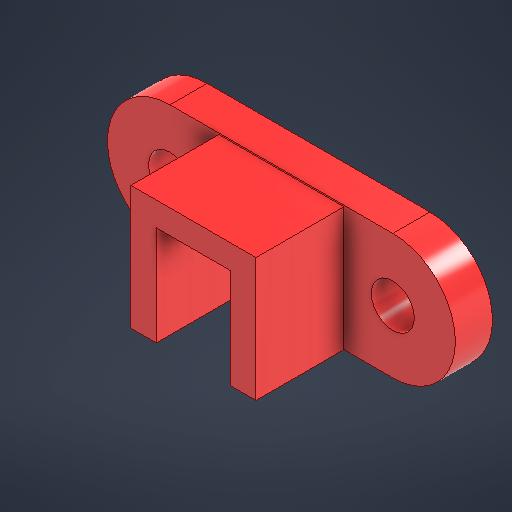
# Autodesk Inventor part: PART 7
Saved by Autodesk Inventor 2026.2 (Build 302298000, 298)
## iProperties
Created: 2026-03-26
Part Number: PART 7
Material: Nylon 6/6
Document SubType Name: Modeling
Designer: LENOVO
Density: 1.13 g/cm^3
Appearance: Light Red
Author: LENOVO
Autodesk Inventor part; units mm, degrees
ref_plane "YZ Plane" through (0, 0, 0) normal (1, 0, 0) x (0, 1, 0)
sketch "Sketch1" plane through (0, 0, 0) normal (0, 0, 1) x (1, 0, 0)
  point P0 (0, 0)
sketch "Sketch2" plane through (0, 0, 0) normal (0, 0, 1) x (1, 0, 0)
  line L0 (-53.7332, 0) -> (60.2668, 0) construction
  line L1 (-53.7332, -32) -> (60.2668, -32)
  line L2 (60.2668, 32) -> (-53.7332, 32)
  arc A0 (-53.7332, 32) -> (-53.7332, -32) centre (-53.7332, 0) ccw
  arc A1 (60.2668, -32) -> (60.2668, 32) centre (60.2668, 0) ccw
  point P0 (0, 0)
  point P1 (3.2668, 0)
  dimension "d0" = 32
  dimension "d1" = 32
  dimension "d2" = 114
  constraints: 8 end point, 4 point on circle, 4 tangent, 2 centre point, 1 horizontal, 1 midpoint, 1 parallel
  measures "d0" radius of A1
  measures "d1" radius of A0
  measures "d2" distance of L2.start L2.end
extrude "Extrusion1" add sketch "Sketch2" against normal blind 19
ref_plane "Work Plane1" through (0, 0, 0) normal (0, 0, 1) x (1, 0, 0)
sketch "Sketch3" plane through (0, 0, 0) normal (0, 0, 1) x (1, 0, 0)
  arc A0 (60.2668, -32) -> (60.2668, 32) centre (60.2668, 0) ccw projected
  line L0 (60.2668, -32) -> (-53.7332, -32) projected
  line L1 (-28.7332, -32) -> (-28.7332, 31.3001)
  line L2 (35.2668, -32) -> (35.2668, 31.3001)
  line L3 (-53.7332, -32) -> (60.2668, -32) projected
  line L4 (-15.7332, -32) -> (-15.7332, 19)
  line L5 (22.2668, 19) -> (22.2668, -32)
  line L6 (-15.7332, 19) -> (22.2668, 19)
  line L7 (-28.7332, 31.3001) -> (35.2668, 31.3001)
  line L8 (-53.7332, 32) -> (60.2668, 32) projected
  point P0 (0, 0)
  point P1 (-54.8329, -31.8056)
  point P2 (3.2668, -32)
  point P3 (3.2668, -32)
  point P4 (3.2668, -32)
  point P5 (-15.7332, 32)
  point P6 (20.2211, 31.3001)
  point P7 (3.2668, -32)
  point P8 (3.2668, -32)
  point P9 (22.2668, -32)
  point P10 (3.2668, -32)
  point P11 (3.2668, -32)
  dimension "d6" = 58.0997
  dimension "d7" = 64
  dimension "d12" = 51
  dimension "d17" = 38
  dimension "d18" = 19
  dimension "d19" = 19
  constraints: 12 end point, 5 coincident, 2 parallel, 2 point on line, 2 vertical, 1 midpoint, 1 perpendicular, 8 other
  measures "d6" horizontal distance of point (-54.833, -31.806) point (3.267, -32)
  measures "d7" distance of L2.end L1.end
  measures "d12" distance of L4.end point (-15.733, -32)
  measures "d17" distance of L4.end L5.start
  measures "d18" distance of point (3.267, -32) L4.start
  measures "d19" distance of point (3.267, -32) point (22.267, -32)
extrude "Extrusion2" add sketch "Sketch3" along normal blind 45 contours L0 L5 L6 L4 L1 L7 L2
ref_plane "Work Plane2" through (0, 0, 0) normal (0, 0, 1) x (1, 0, 0)
sketch "Sketch5" plane through (-53.7332, -32, -19) normal (0, -1, 0) x (1, 0, 0)
  line L0 (38, 19) -> (76, 19) projected
  line L1 (38, 19) -> (76, 19)
  line L2 (76, 19) -> (76, 13)
  line L3 (76, 13) -> (38, 13)
  line L4 (38, 13) -> (38, 19)
  point P0 (53.7332, 19)
  dimension "d16" = 38
  dimension "d20" = 6
  constraints: 8 end point, 2 parallel, 1 horizontal, 1 perpendicular
  measures "d16" distance of L2.end L3.end
  measures "d20" distance of L1.end L2.end
extrude "Extrusion3" cut sketch "Sketch5" against normal blind 51
sketch "Sketch6" plane through (-15.7332, -32, 45) normal (1, 0, 0) x (0, 0, -1)
  line L0 (0, 51) -> (51, 51)
  line L1 (51, 51) -> (51, 0)
  line L2 (51, 0) -> (0, 51)
  point P0 (45, 32)
  constraints: 6 end point, 1 perpendicular
extrude "Extrusion4" add sketch "Sketch6" along normal blind 51
sketch "Sketch7" plane through (0, 0, 0) normal (0, 0, 1) x (1, 0, 0)
  line L0 (-28.7332, -32) -> (-28.7332, 31.3001) projected
  line L1 (-28.7332, 31.3001) -> (35.2668, 31.3001) projected
  line L2 (35.2668, 31.3001) -> (35.2668, -32) projected
  line L3 (35.2668, -32) -> (60.2668, -32) projected
  arc A0 (60.2668, -32) -> (60.2668, 32) centre (60.2668, 0) ccw projected
  line L4 (60.2668, 32) -> (-53.7332, 32) projected
  arc A1 (-53.7332, 32) -> (-53.7332, -32) centre (-53.7332, 0) ccw projected
  line L5 (-53.7332, -32) -> (-28.7332, -32) projected
  circle A2 centre (-53.7332, 0) radius 11
  circle A3 centre (60.2668, 0) radius 11
  point P0 (0, 0)
  dimension "d25" = 22
  dimension "d26" = 22
  dimension "d27" = 114
  constraints: 2 centre point, 2 coincident
  measures "d25" diameter of A3
  measures "d26" diameter of A2
  measures "d27" distance of A0.centre A1.centre
extrude "Extrusion5" cut sketch "Sketch7" against normal through all contours A2 | A3
body "Solid1"
